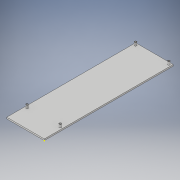
# Autodesk Inventor part: Part1
Saved by Autodesk Inventor 2018 (Build 220112000, 112)
## iProperties
Created: 2020-05-28
Part Number: Part1
Material: Generic
Document SubType Name: Modeling
Designer: Zach
Density: 1 g/cm^3
Appearance: Default
Author: Zach
Autodesk Inventor part; units mm, degrees
ref_plane "YZ Plane" through (0, 0, 0) normal (1, 0, 0) x (0, 1, 0)
ref_plane "XZ Plane" through (0, 0, 0) normal (0, 1, 0) x (-1, 0, 0)
ref_plane "XY Plane" through (0, 0, 0) normal (0, 0, 1) x (1, 0, 0)
sketch "Sketch1" plane through (0, 0, 0) normal (0, 1, 0) x (-1, 0, 0)
  point P0 (0, 0)
sketch "Sketch2" plane through (0, 0, 0) normal (0, 1, 0) x (-1, 0, 0)
  line L0 (0.0816, -0.0238) -> (77.0816, -0.0238)
  line L1 (77.0816, -0.0238) -> (77.0816, -264.0238)
  line L2 (77.0816, -264.0238) -> (0.0816, -264.0238)
  line L3 (0.0816, -264.0238) -> (0.0816, -0.0238)
  line L4 (2.0816, -2.0238) -> (75.0816, -2.0238)
  line L5 (75.0816, -2.0238) -> (75.0816, -262.0238)
  line L6 (75.0816, -262.0238) -> (2.0816, -262.0238)
  line L7 (2.0816, -262.0238) -> (2.0816, -2.0238)
  line L8 (2.0816, -2.0238) -> (2.0816, -4.4588)
  line L9 (75.0816, -2.0238) -> (75.0816, -4.4588)
  line L10 (2.0816, -262.0238) -> (2.0816, -226.5538)
  circle A0 centre (72.3366, -4.2738) radius 2.25
  circle A1 centre (4.3316, -4.4588) radius 2.25
  circle A2 centre (4.3316, -226.5538) radius 2.25
  circle A3 centre (72.3366, -226.5538) radius 2.25
  dimension "d24" = 4.5
  dimension "d25" = 4.5
  dimension "d3" = 77
  dimension "d4" = 264
  dimension "d7" = 73
  dimension "d8" = 260
  dimension "d23" = 4.5
  dimension "d26" = 4.5
  constraints: 22 end point, 4 parallel, 3 point on line, 2 centre point, 2 horizontal, 2 horizontal alignment, 2 perpendicular, 1 tangent, 4 other
  measures "d3" distance of L1.end L2.end
  measures "d4" distance of L0.end L1.end
  measures "d7" distance of L5.end L6.end
  measures "d8" distance of L4.end L5.end
  measures "d23" diameter of A0
  measures "d26" diameter of A3
extrude "Extrusion1" add sketch "Sketch2" along normal blind 3 contours L0 L1 L2 L3 | A1 | A2 | A0 | L4 L5 L6 L7 | A3
sketch "Sketch3" plane through (-77.1633, 3, -264.0476) normal (0, 1, 0) x (1, 0, 0)
  line L0 (2.0816, -2.0238) -> (2.0816, -4.4588)
  line L1 (75.0816, -2.0238) -> (75.0816, -4.4588)
  circle A0 centre (72.3366, -4.2738) radius 2.25
  circle A1 centre (4.3316, -4.4588) radius 2.25
  circle A2 centre (4.3316, -226.5538) radius 2.25
  circle A3 centre (72.3366, -226.5538) radius 2.25
  dimension "d29" = 4.5
  dimension "d30" = 4.5
  dimension "d28" = 4.5
  dimension "d27" = 4.5
  constraints: 4 end point, 3 centre point, 1 horizontal alignment, 2 other
  measures "d30" diameter of A0
  measures "d28" diameter of A2
  measures "d27" diameter of A3
extrude "Extrusion3" add sketch "Sketch3" along normal blind 6
hole "Hole1" at (-4.8266, 9, -259.7738) direction (0, -1, 0) diameter 3 depth 4
hole "Hole2" at (-4.8266, 9, -37.4938) direction (0, -1, 0) diameter 3 depth 4
hole "Hole3" at (-72.8316, 9, -37.4938) direction (0, -1, 0) diameter 3 depth 4
hole "Hole4" at (-72.8316, 9, -259.5888) direction (0, -1, 0) diameter 3 depth 4
body "Solid1"
